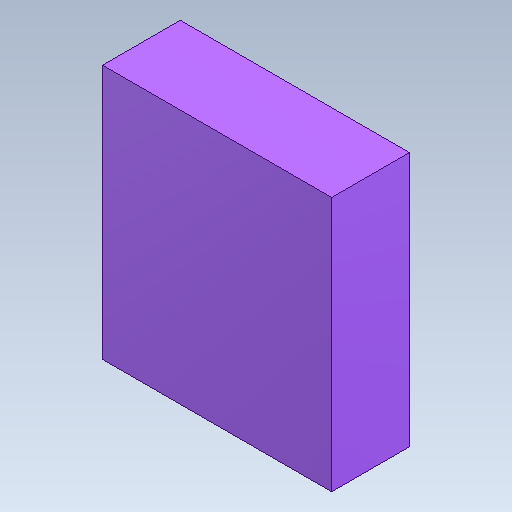
# Autodesk Inventor part: I1_IND_LPS3015
Saved by Autodesk Inventor 2021 (Build 250183000, 183)
## iProperties
Created: 2020-11-03
Part Number: I1_IND_LPS3015
Material: Generic
Document SubType Name: Modeling
Designer: faiya
Density: 1 g/cm^3
Appearance: IND_LPS3015, I1_IND_LPS3015
Author: faiya
Autodesk Inventor part; units mm, degrees
ref_plane "YZ Plane" through (0, 0, 0) normal (1, 0, 0) x (0, 1, 0)
ref_plane "XZ Plane" through (0, 0, 0) normal (0, 1, 0) x (-1, 0, 0)
ref_plane "XY Plane" through (0, 0, 0) normal (0, 0, 1) x (1, 0, 0)
sketch "IND_LPS3015, I1_IND_LPS3015_42" plane through (0, 0, 0) normal (0, 0, 1) x (1, 0, 0)
  line L0 (-1.4732, 1.6002) -> (1.4732, 1.6002)
  line L1 (1.4732, 1.6002) -> (1.4732, -1.6764)
  line L2 (1.4732, -1.6764) -> (-1.4732, -1.6764)
  line L3 (-1.4732, -1.6764) -> (-1.4732, 1.6002)
  constraints: 8 end point
extrude "Extrusion1" add sketch "IND_LPS3015, I1_IND_LPS3015_42" along normal blind 1
body "Solid1"
